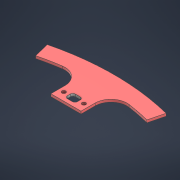
# Autodesk Inventor part: sensor
Saved by Autodesk Inventor 2022 (Build 260153000, 153)
## iProperties
Created: 2021-10-17
Part Number: sensor
Material: 一般
Document SubType Name: Modeling
Designer: shiok
Density: 1 g/cm^3
Appearance: 既定
Author: shiok
Autodesk Inventor part; units mm, degrees
ref_plane "YZ Plane" through (0, 0, 0) normal (1, 0, 0) x (0, 1, 0)
ref_plane "XZ Plane" through (0, 0, 0) normal (0, 1, 0) x (-1, 0, 0)
ref_plane "XY Plane" through (0, 0, 0) normal (0, 0, 1) x (1, 0, 0)
sketch "スケッチ1" plane through (0, 0, 0) normal (0, 1, 0) x (-1, 0, 0)
  arc A0 (0, -152.8163) -> (37.4507, -148.1562) centre (0, 0) ccw
  line L0 (37.4507, -148.1562) -> (0, 0)
  line L1 (0, 0) -> (0, -152.8163)
  arc A1 (9.5, -142.5) -> (35, -138.4612) centre (0, 0) ccw
  line L2 (9.5, -142.5) -> (9.5, -122.5)
  line L3 (9.5, -122.5) -> (0, -122.5)
  arc A2 (-37.4507, -148.1562) -> (0, -152.8163) centre (0, 0) ccw
  line L4 (-37.4507, -148.1562) -> (0, 0)
  arc A3 (-35, -138.4612) -> (-9.5, -142.5) centre (0, 0) ccw
  line L5 (-9.5, -142.5) -> (-9.5, -122.5)
  line L6 (-9.5, -122.5) -> (0, -122.5)
  line L7 (9.5, -142.5) -> (0, -142.5) construction
  line L8 (-9.5, -142.5) -> (0, -142.5) construction
  line L9 (-9.5, -180.2611) -> (-9.5, 6.4286)
  line L10 (9.5, -180.2611) -> (9.5, 6.4286)
  line L11 (0, -130) -> (-3.1667, -130)
  line L12 (-3.1667, -130) -> (-3.1667, -125)
  line L13 (-3.1667, -125) -> (0, -125)
  line L14 (0, -130) -> (3.1667, -130)
  line L15 (3.1667, -130) -> (3.1667, -125)
  line L16 (3.1667, -125) -> (0, -125)
  point P0 (0, -125)
  dimension "d4" = 19
  dimension "d7" = 20
  dimension "d12" = 122.5
  dimension "d13" = 10
  dimension "d29" = 19
  dimension "d31" = 70
  dimension "d32" = 5
  dimension "d33" = 6.3333
  dimension "d34" = 2.5
  constraints: 34 end point, 8 point on circle, 8 symmetric about line, 7 point on line, 4 centre point, 4 coincident, 3 perpendicular, 2 vertical, 1 horizontal, 1 parallel, 2 other
  measures "d4" distance of L2.end L5.end
  measures "d7" distance between parallel lines of L7 L3
  measures "d12" distance from line of point (0, 0) L3
  measures "d13" radial gap between concentric circles of A0 A1
  measures "d29" distance between parallel lines of L9 L10
  measures "d31" distance of A1.end A3.start
  measures "d32" distance of L11.end L12.end
  measures "d33" distance between parallel lines of L15 L12
  measures "d34" distance between parallel lines of L13 L6
extrude "押し出し1" add sketch "スケッチ1" along normal blind 1.6 contours L1 L14 L15 L16 L3 L2 L10 A0 | A2 L9 L5 L6 L1 L13 L12 L11 | L10 A1 L0 A0 | A2 L4 A3 L9
sketch "スケッチ2" plane through (0, 1.6, 0) normal (0, 1, 0) x (1, 0, 0)
  line L0 (9.5, 122.5) -> (9.5, 142.5) projected
  arc A0 (35, 138.4612) -> (9.5, 142.5) centre (0, 0) ccw projected
  line L1 (35, 138.4612) -> (37.4507, 148.1562) projected
  arc A1 (37.4507, 148.1562) -> (-37.4507, 148.1562) centre (0, 0) ccw projected
  line L2 (-37.4507, 148.1562) -> (-35, 138.4612) projected
  arc A2 (-9.5, 142.5) -> (-35, 138.4612) centre (0, 0) ccw projected
  line L3 (-9.5, 142.5) -> (-9.5, 122.5) projected
  line L4 (-9.5, 122.5) -> (9.5, 122.5) projected
  line L5 (-9.5, 122.5) -> (5.5, 122.5)
  line L6 (5.5, 122.5) -> (5.5, 132.5)
  line L7 (5.5, 132.5) -> (-9.5, 132.5)
  line L8 (-9.5, 132.5) -> (-9.5, 122.5)
  line L9 (-6.3333, 127.5) -> (-3.1667, 127.5) construction
  line L10 (-6.3333, 127.5) -> (-9.5, 127.5) construction
  line L11 (-3.1667, 125) -> (-3.1667, 130) projected
  point P0 (6.3333, 127.5)
  dimension "d19" = 10
  dimension "d20" = 15
  constraints: 12 end point, 2 collinear, 2 parallel, 1 horizontal, 1 midpoint, 1 perpendicular, 2 other
  measures "d19" distance of L6.end L5.end
  measures "d20" distance of L6.end L7.end
hole "穴1" at (6.3333, 1.6, -127.5) at (-6.3333, 1.6, -127.5) direction (0, -1, 0) diameter 2.4 depth 1.6 tip angle 118 clearance for "Countersunk Flat Head Screw ISO 2009/7046" size "M2" standard "ISO"
fillet "フィレット1" radius 10 2 edges at (9.5, 0.8, -142.5) (-9.5, 0.8, -142.5)
fillet "フィレット2" radius 1.5 4 edges at (-3.1667, 0.8, -130) (3.1667, 0.8, -125) (3.1667, 0.8, -130) (-3.1667, 0.8, -125)
